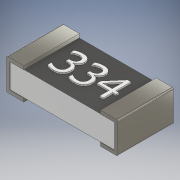
# Autodesk Inventor part: 21-1001
Saved by Autodesk Inventor 2018 (Build 220112000, 112)
## iProperties
Created: 2019-09-21
Part Number: 21-1001
Material: Copper
Document SubType Name: Modeling
Designer: Bradley
Density: 8.94 g/cm^3
Appearance: Smooth - White
Author: Bradley
Autodesk Inventor part; units mm, degrees
ref_plane "YZ Plane" through (0, 0, 0) normal (1, 0, 0) x (0, 1, 0)
ref_plane "XZ Plane" through (0, 0, 0) normal (0, 1, 0) x (-1, 0, 0)
ref_plane "XY Plane" through (0, 0, 0) normal (0, 0, 1) x (1, 0, 0)
sketch "Sketch1" plane through (0, 0, 0) normal (0, 1, 0) x (-1, 0, 0)
  line L0 (0.75, 0.175) -> (-0.75, 0.175)
  line L1 (-0.75, 0.175) -> (-0.75, -0.175)
  line L2 (-0.75, -0.175) -> (0.75, -0.175)
  line L3 (0.75, -0.175) -> (0.75, 0.175)
  line L4 (0.55, 0.175) -> (0.55, 0.225)
  line L5 (0.55, 0.225) -> (0.8, 0.225)
  line L6 (0.8, 0.225) -> (0.8, -0.225)
  line L7 (0.8, -0.225) -> (0.55, -0.225)
  line L8 (0.55, -0.225) -> (0.55, -0.175)
  line L9 (-0.55, 0.175) -> (-0.55, 0.225)
  line L10 (-0.55, 0.225) -> (-0.8, 0.225)
  line L11 (-0.8, 0.225) -> (-0.8, -0.225)
  line L12 (-0.8, -0.225) -> (-0.55, -0.225)
  line L13 (-0.55, -0.175) -> (-0.55, -0.225)
  line L14 (0.55, 0.175) -> (-0.55, 0.175)
  point P0 (0, 0)
  point P1 (0, 0.175)
  point P2 (0.75, 0)
  dimension "d0" = 1.6
  dimension "d1" = 0.05
  dimension "d2" = 0.05
  dimension "d3" = 0.45
  dimension "d4" = 0.25
  constraints: 30 end point, 12 point on line, 7 perpendicular, 3 collinear, 3 midpoint, 2 parallel, 1 horizontal, 1 horizontal alignment, 1 vertical, 1 vertical alignment
  measures "d0" distance between parallel lines of L11 L6
  measures "d1" distance of L7.end L8.end
  measures "d2" distance between parallel lines of L6 L3
  measures "d3" distance of L5.end L6.end
  measures "d4" distance of L6.end L7.end
extrude "Extrusion1" add sketch "Sketch1" along normal mid plane 0.8 contours L0 L4 L5 L6 L7 L8 L2 L3 | L0 L1 L2 L13 L12 L11 L10 L9
extrude "Extrusion2" add sketch "Sketch1" along normal mid plane 0.79 contours L3 L2 L1 L0
sketch "Sketch2" plane through (-0.55, -0.395, 0.175) normal (0, 0, 1) x (1, 0, 0)
  line L0 (0, 0) -> (0, 0.79) projected
  line L1 (1.1, 0) -> (0, 0) projected
  line L2 (1.1, 0) -> (1.1, 0.79) projected
  line L3 (0, 0.79) -> (1.1, 0.79) projected
  line L4 (0, 0.395) -> (1.1, 0.395) construction
  spline S0 degree 2 poles (0.2369, 0.5571) (0.2223, 0.5571) (0.1934, 0.5499) (0.1795, 0.5444) knots 0 0 0 1 2 2 2
  spline S1 degree 2 poles (0.1795, 0.5444) (0.1665, 0.5389) (0.1474, 0.5273) (0.14, 0.5221) knots 0 0 0 1 2 2 2
  line L5 (0.14, 0.5221) -> (0.1367, 0.5221)
  line L6 (0.1367, 0.5221) -> (0.1367, 0.5788)
  spline S2 degree 2 poles (0.1367, 0.5788) (0.1542, 0.5882) (0.2142, 0.6034) (0.2411, 0.6034) knots 0 0 0 1 2 2 2
  spline S3 degree 2 poles (0.2411, 0.6034) (0.2683, 0.6034) (0.3088, 0.5924) (0.3254, 0.5807) knots 0 0 0 1 2 2 2
  spline S4 degree 2 poles (0.3254, 0.5807) (0.3429, 0.5681) (0.361, 0.5315) (0.361, 0.5068) knots 0 0 0 1 2 2 2
  spline S5 degree 2 poles (0.361, 0.5068) (0.361, 0.4738) (0.3176, 0.4238) (0.2871, 0.4174) knots 0 0 0 1 2 2 2
  line L7 (0.2871, 0.4174) -> (0.2871, 0.4135)
  spline S6 degree 2 poles (0.2871, 0.4135) (0.2998, 0.4109) (0.3286, 0.3992) (0.3409, 0.3875) knots 0 0 0 1 2 2 2
  spline S7 degree 2 poles (0.3409, 0.3875) (0.3532, 0.3762) (0.3688, 0.3399) (0.3688, 0.3136) knots 0 0 0 1 2 2 2
  spline S8 degree 2 poles (0.3688, 0.3136) (0.3688, 0.2867) (0.3503, 0.241) (0.3335, 0.2235) knots 0 0 0 1 2 2 2
  spline S9 degree 2 poles (0.3335, 0.2235) (0.316, 0.2054) (0.2664, 0.1866) (0.2349, 0.1866) knots 0 0 0 1 2 2 2
  spline S10 degree 2 poles (0.2349, 0.1866) (0.2048, 0.1866) (0.1458, 0.2012) (0.1257, 0.2112) knots 0 0 0 1 2 2 2
  line L8 (0.1257, 0.2112) -> (0.1257, 0.2679)
  line L9 (0.1257, 0.2679) -> (0.1296, 0.2679)
  spline S11 degree 2 poles (0.1296, 0.2679) (0.1464, 0.2556) (0.2035, 0.2329) (0.2317, 0.2329) knots 0 0 0 1 2 2 2
  spline S12 degree 2 poles (0.2317, 0.2329) (0.2482, 0.2329) (0.2813, 0.2433) (0.2923, 0.2553) knots 0 0 0 1 2 2 2
  spline S13 degree 2 poles (0.2923, 0.2553) (0.303, 0.2673) (0.3143, 0.2958) (0.3143, 0.3175) knots 0 0 0 1 2 2 2
  spline S14 degree 2 poles (0.3143, 0.3175) (0.3143, 0.3392) (0.3017, 0.3674) (0.2904, 0.3756) knots 0 0 0 1 2 2 2
  spline S15 degree 2 poles (0.2904, 0.3756) (0.279, 0.3837) (0.2482, 0.3898) (0.2301, 0.3898) knots 0 0 0 1 2 2 2
  line L10 (0.2301, 0.3898) -> (0.2074, 0.3898)
  line L11 (0.2074, 0.3898) -> (0.2074, 0.4342)
  line L12 (0.2074, 0.4342) -> (0.2252, 0.4342)
  spline S16 degree 2 poles (0.2252, 0.4342) (0.2612, 0.4342) (0.3066, 0.4686) (0.3066, 0.5013) knots 0 0 0 1 2 2 2
  spline S17 degree 2 poles (0.3066, 0.5013) (0.3066, 0.5166) (0.2949, 0.5383) (0.2855, 0.5448) knots 0 0 0 1 2 2 2
  spline S18 degree 2 poles (0.2855, 0.5448) (0.2754, 0.5516) (0.2508, 0.5571) (0.2369, 0.5571) knots 0 0 0 1 2 2 2
  spline S19 degree 2 poles (0.537, 0.5571) (0.5224, 0.5571) (0.4936, 0.5499) (0.4797, 0.5444) knots 0 0 0 1 2 2 2
  spline S20 degree 2 poles (0.4797, 0.5444) (0.4667, 0.5389) (0.4476, 0.5273) (0.4401, 0.5221) knots 0 0 0 1 2 2 2
  line L13 (0.4401, 0.5221) -> (0.4369, 0.5221)
  line L14 (0.4369, 0.5221) -> (0.4369, 0.5788)
  spline S21 degree 2 poles (0.4369, 0.5788) (0.4544, 0.5882) (0.5143, 0.6034) (0.5412, 0.6034) knots 0 0 0 1 2 2 2
  spline S22 degree 2 poles (0.5412, 0.6034) (0.5685, 0.6034) (0.609, 0.5924) (0.6255, 0.5807) knots 0 0 0 1 2 2 2
  spline S23 degree 2 poles (0.6255, 0.5807) (0.643, 0.5681) (0.6612, 0.5315) (0.6612, 0.5068) knots 0 0 0 1 2 2 2
  spline S24 degree 2 poles (0.6612, 0.5068) (0.6612, 0.4738) (0.6177, 0.4238) (0.5873, 0.4174) knots 0 0 0 1 2 2 2
  line L15 (0.5873, 0.4174) -> (0.5873, 0.4135)
  spline S25 degree 2 poles (0.5873, 0.4135) (0.5999, 0.4109) (0.6288, 0.3992) (0.6411, 0.3875) knots 0 0 0 1 2 2 2
  spline S26 degree 2 poles (0.6411, 0.3875) (0.6534, 0.3762) (0.669, 0.3399) (0.669, 0.3136) knots 0 0 0 1 2 2 2
  spline S27 degree 2 poles (0.669, 0.3136) (0.669, 0.2867) (0.6505, 0.241) (0.6336, 0.2235) knots 0 0 0 1 2 2 2
  spline S28 degree 2 poles (0.6336, 0.2235) (0.6161, 0.2054) (0.5665, 0.1866) (0.5351, 0.1866) knots 0 0 0 1 2 2 2
  spline S29 degree 2 poles (0.5351, 0.1866) (0.5049, 0.1866) (0.4459, 0.2012) (0.4259, 0.2112) knots 0 0 0 1 2 2 2
  line L16 (0.4259, 0.2112) -> (0.4259, 0.2679)
  line L17 (0.4259, 0.2679) -> (0.4297, 0.2679)
  spline S30 degree 2 poles (0.4297, 0.2679) (0.4466, 0.2556) (0.5036, 0.2329) (0.5318, 0.2329) knots 0 0 0 1 2 2 2
  spline S31 degree 2 poles (0.5318, 0.2329) (0.5484, 0.2329) (0.5814, 0.2433) (0.5925, 0.2553) knots 0 0 0 1 2 2 2
  spline S32 degree 2 poles (0.5925, 0.2553) (0.6032, 0.2673) (0.6145, 0.2958) (0.6145, 0.3175) knots 0 0 0 1 2 2 2
  spline S33 degree 2 poles (0.6145, 0.3175) (0.6145, 0.3392) (0.6019, 0.3674) (0.5905, 0.3756) knots 0 0 0 1 2 2 2
  spline S34 degree 2 poles (0.5905, 0.3756) (0.5792, 0.3837) (0.5484, 0.3898) (0.5302, 0.3898) knots 0 0 0 1 2 2 2
  line L18 (0.5302, 0.3898) -> (0.5075, 0.3898)
  line L19 (0.5075, 0.3898) -> (0.5075, 0.4342)
  line L20 (0.5075, 0.4342) -> (0.5254, 0.4342)
  spline S35 degree 2 poles (0.5254, 0.4342) (0.5613, 0.4342) (0.6067, 0.4686) (0.6067, 0.5013) knots 0 0 0 1 2 2 2
  spline S36 degree 2 poles (0.6067, 0.5013) (0.6067, 0.5166) (0.5951, 0.5383) (0.5857, 0.5448) knots 0 0 0 1 2 2 2
  spline S37 degree 2 poles (0.5857, 0.5448) (0.5756, 0.5516) (0.551, 0.5571) (0.537, 0.5571) knots 0 0 0 1 2 2 2
  line L21 (0.9866, 0.3324) -> (0.939, 0.3324)
  line L22 (0.939, 0.3324) -> (0.939, 0.195)
  line L23 (0.939, 0.195) -> (0.8874, 0.195)
  line L24 (0.8874, 0.195) -> (0.8874, 0.3324)
  line L25 (0.8874, 0.3324) -> (0.7108, 0.3324)
  line L26 (0.7108, 0.3324) -> (0.7108, 0.3888)
  line L27 (0.7108, 0.3888) -> (0.8897, 0.595)
  line L28 (0.8897, 0.595) -> (0.939, 0.595)
  line L29 (0.939, 0.595) -> (0.939, 0.3756)
  line L30 (0.939, 0.3756) -> (0.9866, 0.3756)
  line L31 (0.9866, 0.3756) -> (0.9866, 0.3324)
  line L32 (0.8874, 0.3756) -> (0.8874, 0.5318)
  line L33 (0.8874, 0.5318) -> (0.7529, 0.3756)
  line L34 (0.7529, 0.3756) -> (0.8874, 0.3756)
  point P0 (0.55, 0.395)
  constraints: 2 end point, 2 midpoint, 1 horizontal
extrude "Extrusion3" add sketch "Sketch2" along normal blind 0.02 contours S0 S1 L5 L6 S2 S3 S4 S5 L7 S6 S7 S8 S9 S10 L8 L9 S11 S12 S13 S14 S15 L10 L11 L12 S16 S17 S18 | S19 S20 L13 L14 S21 S22 S23 S24 L15 S25 S26 S27 S28 S29 L16 L17 S30 S31 S32 S33 S34 L18 L19 L20 S35 S36 S37 | L21 L22 L23 L24 L25 L26 L27 L28 L29 L30 L31
fillet "Fillet1" radius 0.02 4 edges at (-0.8, 0, 0.225) (-0.8, 0, -0.225) (0.8, 0, 0.225) (0.8, 0, -0.225)
equation "\"d2\" = d1"
body "Solid1"
